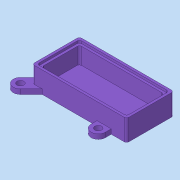
# Autodesk Inventor part: BackupNanoCasePart1
Saved by Autodesk Inventor 2017 (Build 210142000, 142)
## iProperties
Created: 2018-02-21
Part Number: BackupNanoCasePart1
Material: ABS Plastic
Document SubType Name: Modeling
Designer: Derek Wider
Density: 1.06 g/cm^3
Appearance: Violet
Author: Derek Wider
Autodesk Inventor part; units mm, degrees
ref_plane "YZ Plane" through (0, 0, 0) normal (1, 0, 0) x (0, 1, 0)
ref_plane "XZ Plane" through (0, 0, 0) normal (0, 1, 0) x (-1, 0, 0)
ref_plane "XY Plane" through (0, 0, 0) normal (0, 0, 1) x (1, 0, 0)
sketch "Sketch1" plane through (0, 0, 0) normal (0, 1, 0) x (-1, 0, 0)
  line L0 (0, 0) -> (50.8, 0)
  line L1 (50.8, 0) -> (50.8, -25.4)
  line L2 (50.8, -25.4) -> (0, -25.4)
  line L3 (0, -25.4) -> (0, 0)
  line L4 (48.26, -22.86) -> (48.26, -2.54)
  line L5 (48.26, -2.54) -> (2.54, -2.54)
  line L6 (2.54, -2.54) -> (2.54, -22.86)
  line L7 (2.54, -22.86) -> (48.26, -22.86)
  dimension "d0" = 50.8
  dimension "d1" = 25.4
  dimension "d2" = 2.54
  constraints: 16 end point, 4 parallel, 2 perpendicular, 1 horizontal, 3 other
  measures "d0" distance of L1.end L2.end
  measures "d1" distance of L0.end L1.end
  measures "d2" distance between parallel lines of L1 L4
extrude "Extrusion1" add sketch "Sketch1" along normal blind 11.43
extrude "Extrusion2" add sketch "Sketch1" along normal blind 1.27 contours L7 L6 L5 L4
sketch "Sketch2" plane through (0, 11.43, 0) normal (0, 1, 0) x (1, 0, 0)
  line L0 (-48.26, 22.86) -> (-2.54, 22.86) projected
  line L1 (-2.54, 22.86) -> (-2.54, 2.54) projected
  line L2 (-2.54, 2.54) -> (-48.26, 2.54) projected
  line L3 (-48.26, 2.54) -> (-48.26, 22.86) projected
  line L4 (-50.8, 0) -> (0, 0) projected
  line L5 (0, 0) -> (0, 25.4) projected
  line L6 (0, 25.4) -> (-50.8, 25.4) projected
  line L7 (-50.8, 25.4) -> (-50.8, 0) projected
  line L8 (-49.53, 24.13) -> (-1.27, 24.13)
  line L9 (-1.27, 24.13) -> (-1.27, 1.27)
  line L10 (-1.27, 1.27) -> (-49.53, 1.27)
  line L11 (-49.53, 1.27) -> (-49.53, 24.13)
  dimension "d7" = 1.27
  constraints: 8 end point, 3 other
  measures "d7" distance between parallel lines of L3 L11
extrude "Extrusion3" cut sketch "Sketch2" against normal blind 1.27 contours L8 L9 L10 L11
fillet "Fillet1" radius 1.27 12 edges at (-2.54, 5.715, -2.54) (-1.27, 10.795, -1.27) (0, 5.715, 0) (-50.8, 5.715, 0) (-49.53, 10.795, -1.27) (-48.26, 5.715, -2.54) (-50.8, 5.715, -25.4) (-49.53, 10.795, -24.13) (-48.26, 5.715, -22.86) (0, 5.715, -25.4) (-1.27, 10.795, -24.13) (-2.54, 5.715, -22.86)
sketch "Sketch3" plane through (0, 0, 0) normal (0, -1, 0) x (1, 0, 0)
  circle A0 centre (-53.975, 3.175) radius 1.8415
  circle A1 centre (-12.065, 3.175) radius 1.8415
  circle A2 centre (-53.975, 3.175) radius 3.81
  circle A3 centre (-12.065, 3.175) radius 3.81
  line L0 (-1.27, 0) -> (-49.53, 0) projected
  line L1 (-56.6691, 0.4809) -> (-50.8, -5.3882)
  line L2 (-51.2809, 5.8691) -> (-45.4118, 0)
  line L3 (-15.8678, 2.941) -> (-15.8678, 0)
  line L4 (-8.255, 3.175) -> (-8.255, 0)
  arc A4 (-1.27, -25.4) -> (0, -24.13) centre (-1.27, -24.13) ccw projected
  line L5 (0, -24.13) -> (0, -1.27) projected
  arc A5 (0, -1.27) -> (-1.27, 0) centre (-1.27, -1.27) ccw projected
  line L6 (-1.27, 0) -> (-49.53, 0) projected
  arc A6 (-49.53, 0) -> (-50.8, -1.27) centre (-49.53, -1.27) ccw projected
  line L7 (-50.8, -1.27) -> (-50.8, -24.13) projected
  arc A7 (-50.8, -24.13) -> (-49.53, -25.4) centre (-49.53, -24.13) ccw projected
  line L8 (-49.53, -25.4) -> (-1.27, -25.4) projected
  line L9 (-50.8, -24.13) -> (-50.8, -1.27) projected
  line L10 (-50.8, -5.3882) -> (-50.8, -1.27)
  arc A8 (-49.53, 0) -> (-50.8, -1.27) centre (-49.53, -1.27) ccw
  line L11 (-49.53, 0) -> (-45.4118, 0)
  point P0 (0, 0)
  dimension "d11" = 3.683
  dimension "d13" = 41.91
  dimension "d14" = 7.62
  dimension "d16" = 3.175
  dimension "d17" = 45
  constraints: 12 end point, 6 point on circle, 5 centre point, 3 equal radius, 3 point on line, 3 tangent, 2 coincident, 2 collinear, 2 perpendicular, 1 horizontal alignment, 1 parallel
  measures "d11" diameter of A0
  measures "d13" distance of A0.centre A1.centre
  measures "d14" diameter of A2
  measures "d16" distance from line of L0 A0.centre
  measures "d17" angle of L0 L2
extrude "Extrusion4" add sketch "Sketch3" against normal blind 2.54 contours A2 | A2 L2 L0 A6 L7 L1 | L3 A3 L0 | A3 L0 | A3 L4 L0 picked at (-11.991, 0.449)
body "Solid1"
